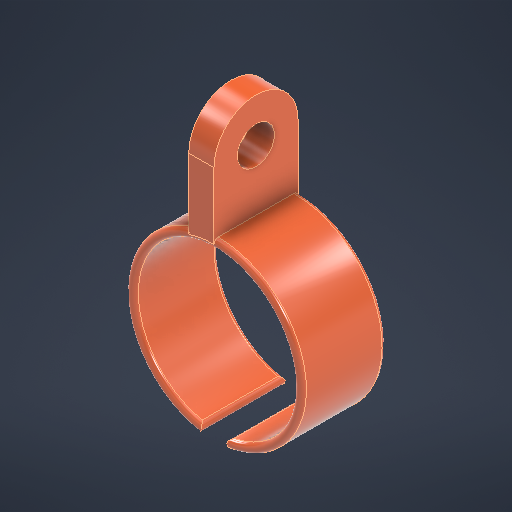
# Autodesk Inventor part: Anillo_Dedos
Saved by Autodesk Inventor 2027 (Build 310192060, 192F)
## iProperties
Created: 2026-06-12
Part Number: Anillo_Dedos
Material: Genérico
Document SubType Name: Modeling
Designer: angel
Density: 1 g/cm^3
Appearance: Suave - Naranja claro
Author: angel
Autodesk Inventor part; units mm, degrees
ref_plane "YZ Plane" through (0, 0, 0) normal (1, 0, 0) x (0, 1, 0)
ref_plane "XZ Plane" through (0, 0, 0) normal (0, 1, 0) x (-1, 0, 0)
ref_plane "XY Plane" through (0, 0, 0) normal (0, 0, 1) x (1, 0, 0)
sketch "Boceto1" plane through (0, 0, 0) normal (0, 0, 1) x (1, 0, 0)
  circle A0 centre (0, -5) radius 10.5
  circle A1 centre (0, -5) radius 9.5
  line L0 (0, 5.5) -> (0, 20.5)
  line L1 (0, 20.5) -> (-3, 20.5)
  line L2 (-3, 20.5) -> (-3, 5.0623)
  line L3 (0, -14.5) -> (1.5, -14.5)
  line L4 (1.5, -14.5) -> (-1.5, -14.5)
  line L5 (-1.5, -14.5) -> (-1.5, -14.3808)
  line L6 (-1.5, -15.5846) -> (-1.5, -14.5)
  line L7 (-1.5, -15.5846) -> (1.5, -15.5846)
  line L8 (1.5, -15.5846) -> (1.5, -14.3808)
  point P0 (0, 0)
  point P1 (-1.5, -15.3923)
  point P2 (1.5, -15.3923)
  dimension "d1" = 19
  dimension "d8" = 21
  dimension "d9" = 15
  dimension "d10" = 3
  dimension "d13" = 1.5
  dimension "d14" = 3
  constraints: 18 end point, 5 point on circle, 3 horizontal, 3 perpendicular, 2 centre point, 2 point on line, 1 coincident, 1 collinear, 1 tangent, 1 vertical
  measures "d1" diameter of A1
  measures "d8" diameter of A0
  measures "d9" distance of L0.start L0.end
  measures "d10" distance of L0.end L1.end
  measures "d13" distance of L3.start L3.end
  measures "d14" distance of L3.end L4.end
extrude "Extrusión1" add sketch "Boceto1" against normal blind 10 contours A0 L8 A1 L5 L6 | A0 L2 L1 L0
sketch "Boceto2" plane through (0, 5.5, 0) normal (1, 0, 0) x (0, 0, -1)
  line L0 (0, 15) -> (10, 15) projected
  line L1 (0, 0) -> (10, 0)
  line L2 (10, 0) -> (10, 15)
  line L3 (10, 15) -> (0, 15)
  line L4 (0, 15) -> (0, 0)
  line L5 (5, 0) -> (5, 5)
  line L6 (5, 5) -> (5, 15)
  line L7 (5, 5) -> (5, 9.4)
  line L8 (5, 9.4) -> (5, 7.2)
  circle A0 centre (5, 7.2) radius 2.2
  line L9 (5, 9.4) -> (5, 12.4)
  line L10 (5, 12.4) -> (10, 12.4)
  line L11 (0, 12.4) -> (5, 12.4)
  point P0 (0, -5.5)
  dimension "d16" = 15
  dimension "d17" = 10
  dimension "d18" = 5
  dimension "d19" = 4.4
  dimension "d22" = 3
  constraints: 22 end point, 5 point on line, 3 equal length, 3 midpoint, 2 perpendicular, 1 coincident, 1 horizontal, 1 vertical, 1 vertical alignment, 2 other
  measures "d16" distance of L1.end L0.end
  measures "d17" distance of L0.start L0.end
  measures "d18" distance of L5.start L5.end
  measures "d19" distance of L5.end L7.end
  measures "d22" distance of L7.end L9.end
extrude "Extrusión2" cut sketch "Boceto2" against normal blind 10 contours L0 L6 L11 L4 | L0 L2 L10 L6 | A0 L6 | L6 A0
fillet "Empalme1" radius 5 2 edges at (-1.5, 17.9, 0) (-1.5, 17.9, -10)
fillet "Empalme2" radius 0.5 10 edges at (10.473, -4.2481, 0) (-10.4719, -5.7679, 0) (0, 4.5, 0) (10.473, -4.2481, -10) (-10.4719, -5.7679, -10) (0, 4.5, -10) (-1.5, -14.3808, -5) (1.5, -14.3808, -5) (-1.5, -15.3923, -5) (1.5, -15.3923, -5)
